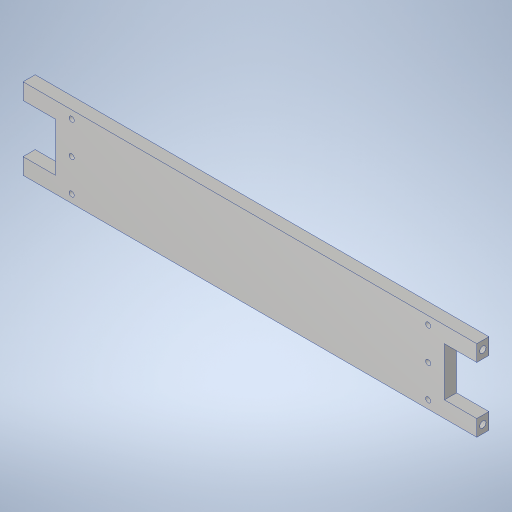
# Autodesk Inventor part: EL2-003
Saved by Autodesk Inventor 2023.4 (Build 274418000, 418)
## iProperties
Created: 2025-01-10
Part Number: EL2-003
Material: Aluminum 6061
Document SubType Name: Modeling
Designer: mavericks
Density: 2.7 g/cm^3
Appearance: Aluminum - Flat
Author: mavericks
Autodesk Inventor part; units mm, degrees
ref_plane "YZ Plane" through (0, 0, 0) normal (1, 0, 0) x (0, 1, 0)
ref_plane "XZ Plane" through (0, 0, 0) normal (0, 1, 0) x (-1, 0, 0)
ref_plane "XY Plane" through (0, 0, 0) normal (0, 0, 1) x (1, 0, 0)
sketch "Sketch1" plane through (0, 0, 0) normal (0, 0, 1) x (1, 0, 0)
  line L0 (-177.8, -31.75) -> (177.8, -31.75)
  line L1 (177.8, -31.75) -> (177.8, 31.75)
  line L2 (177.8, 31.75) -> (-177.8, 31.75)
  line L3 (-177.8, 31.75) -> (-177.8, -31.75)
  line L4 (-177.8, -31.75) -> (177.8, 31.75) construction
  line L5 (177.8, -31.75) -> (-177.8, 31.75) construction
  point P0 (0, 0)
  dimension "d0" = 355.6
  dimension "d1" = 63.5
  constraints: 12 end point, 2 midpoint, 2 parallel, 1 horizontal, 1 perpendicular
  measures "d0" distance of L2.end L1.end
  measures "d1" distance of L1.end L0.end
extrude "Extrusion1" add sketch "Sketch1" along normal blind 9.525
sketch "Sketch4" plane through (0, 0, 9.525) normal (0, 0, 1) x (1, 0, 0)
  line L0 (-139.7, 0) -> (139.7, 0) construction
  point P0 (0, 0)
  point P1 (-139.7, 25.4)
  point P2 (-139.7, -25.4)
  point P3 (139.7, 25.4)
  point P4 (139.7, -25.4)
  point P5 (0, 0)
  dimension "d19" = 25.4
  dimension "d20" = 25.4
  dimension "d21" = 279.4
  constraints: 4 horizontal alignment, 4 vertical alignment, 2 end point, 1 coincident, 1 horizontal, 1 midpoint
  measures "d19" distance of L0.start point (-139.7, 25.4)
  measures "d20" distance of point (-139.7, -25.4) L0.start
  measures "d21" distance of L0.start L0.end
hole "Hole2" at (-139.7, 25.4, 9.525) at (-139.7, 0, 9.525) at (-139.7, -25.4, 9.525) at (139.7, 25.4, 9.525) at (139.7, 0, 9.525) at (139.7, -25.4, 9.525) direction (0, 0, -1) diameter 3.9624 end through all thread size "10-32 UNF" class "2B" standard "ANSI Unified Screw Threads"
sketch "Sketch5" plane through (177.8, -31.75, 0) normal (1, 0, 0) x (0, 0, -1)
  line L0 (0, 63.5) -> (-9.525, 63.5) construction
  line L1 (-4.7625, 57.15) -> (-4.7625, 6.35) construction
  line L2 (0, 0) -> (0, 63.5) construction
  point P0 (0, 31.75)
  point P1 (-4.7625, 63.5)
  point P2 (-4.7625, 31.75)
  point P3 (0, 31.75)
  dimension "d29" = 50.8
  constraints: 3 midpoint, 2 end point, 2 vertical alignment, 1 horizontal alignment, 1 vertical
  measures "d29" distance of L1.start L1.end
hole "Hole3" at (177.8, 25.4, 4.7625) at (177.8, -25.4, 4.7625) direction (-1, 0, 0) diameter 4.9784 depth 25.4 tip angle 118 thread size "1/4-20 UNC" class "2B" standard "ANSI Unified Screw Threads"
sketch "Sketch6" plane through (-177.8, -31.75, 0) normal (-1, 0, 0) x (0, 0, 1)
  line L0 (0, 63.5) -> (9.525, 63.5) construction
  line L1 (4.7625, 57.15) -> (4.7625, 6.35) construction
  point P0 (0, 31.75)
  point P1 (4.7625, 63.5)
  point P2 (4.7625, 31.75)
  dimension "d37" = 50.8
  constraints: 2 end point, 2 midpoint, 2 vertical alignment, 1 horizontal alignment, 1 vertical
  measures "d37" distance of L1.start L1.end
hole "Hole4" at (-177.8, 25.4, 4.7625) at (-177.8, -25.4, 4.7625) direction (1, 0, 0) diameter 4.3434 depth 25.4 tip angle 118 thread size "12-24 UNC" class "2B" standard "ANSI Unified Screw Threads"
sketch "Sketch8" plane through (0, 0, 9.525) normal (0, 0, 1) x (1, 0, 0)
  line L0 (-152.4, 19.05) -> (-177.8, 19.05)
  line L1 (-177.8, 19.05) -> (-177.8, -19.05)
  line L2 (-177.8, -19.05) -> (-152.4, -19.05)
  line L3 (-152.4, -19.05) -> (-152.4, 19.05)
  line L4 (-152.4, 19.05) -> (-177.8, -19.05) construction
  line L5 (-177.8, 19.05) -> (-152.4, -19.05) construction
  line L6 (177.8, 31.75) -> (-177.8, 31.75) projected
  line L7 (-177.8, 31.75) -> (-177.8, -31.75) projected
  line L8 (177.8, 19.05) -> (152.4, 19.05)
  line L9 (152.4, 19.05) -> (152.4, -19.05)
  line L10 (152.4, -19.05) -> (177.8, -19.05)
  line L11 (177.8, -19.05) -> (177.8, 19.05)
  line L12 (177.8, 19.05) -> (152.4, -19.05) construction
  line L13 (152.4, 19.05) -> (177.8, -19.05) construction
  line L14 (177.8, -31.75) -> (177.8, 31.75) projected
  point P0 (0, 0)
  point P1 (-165.1, 0)
  point P2 (165.1, 0)
  dimension "d45" = 25.4
  dimension "d46" = 38.1
  dimension "d47" = 12.7
  dimension "d49" = 25.4
  dimension "d50" = 38.1
  dimension "d52" = 12.7
  constraints: 24 end point, 4 midpoint, 4 parallel, 2 horizontal, 2 perpendicular, 2 point on line
  measures "d45" distance of L2.end L1.end
  measures "d46" distance of L0.end L1.end
  measures "d47" distance between parallel lines of L6 L0
  measures "d49" distance of L10.end L9.end
  measures "d50" distance of L9.end L8.end
  measures "d52" distance between parallel lines of L6 L8
extrude "Extrusion3" cut sketch "Sketch8" against normal blind 39.6875
body "Solid1"
